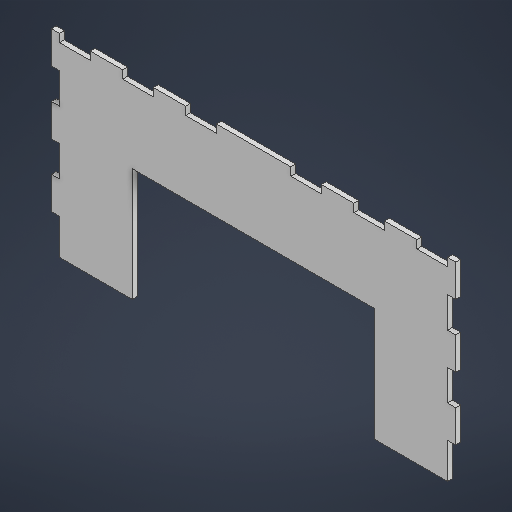
# Autodesk Inventor part: Part1
Saved by Autodesk Inventor 2027.1 (Build 311270010, 270A)
## iProperties
Created: 2026-10-07
Part Number: Part1
Material: Generic
Document SubType Name: Modeling
Designer: daniel
Density: 1 g/cm^3
Appearance: Default
Author: daniel
Autodesk Inventor part; units mm, degrees
ref_plane "YZ Plane" through (0, 0, 0) normal (1, 0, 0) x (0, 1, 0)
ref_plane "XZ Plane" through (0, 0, 0) normal (0, 1, 0) x (-1, 0, 0)
ref_plane "XY Plane" through (0, 0, 0) normal (0, 0, 1) x (1, 0, 0)
sketch "Sketch1" plane through (0, 0, 0) normal (0, 0, 1) x (1, 0, 0)
  line L0 (-39.6936, 53.8926) -> (210.3064, 53.8926)
  line L1 (210.3064, 53.8926) -> (210.3064, -66.1074)
  line L2 (210.3064, -66.1074) -> (-39.6936, -66.1074)
  line L3 (-39.6936, -66.1074) -> (-39.6936, 53.8926)
  line L4 (78.3064, 19.8926) -> (92.3064, 19.8926)
  line L5 (92.3064, 19.8926) -> (92.3064, 14.8926)
  line L6 (92.3064, 14.8926) -> (78.3064, 14.8926)
  line L7 (78.3064, 14.8926) -> (78.3064, 19.8926)
  line L8 (70.3064, 43.8926) -> (75.3064, 43.8926)
  line L9 (75.3064, 43.8926) -> (75.3064, 29.8926)
  line L10 (75.3064, 29.8926) -> (70.3064, 29.8926)
  line L11 (70.3064, 29.8926) -> (70.3064, 43.8926)
  line L12 (95.3064, 43.8926) -> (100.3064, 43.8926)
  line L13 (100.3064, 43.8926) -> (100.3064, 29.8926)
  line L14 (100.3064, 29.8926) -> (95.3064, 29.8926)
  line L15 (95.3064, 29.8926) -> (95.3064, 43.8926)
  line L16 (10.3064, -66.1074) -> (160.3064, -66.1074)
  line L17 (160.3064, -66.1074) -> (160.3064, 3.8926)
  line L18 (160.3064, 3.8926) -> (10.3064, 3.8926)
  line L19 (10.3064, 3.8926) -> (10.3064, -66.1074)
  line L20 (-39.6936, 53.8926) -> (-34.6936, 53.8926)
  line L21 (-34.6936, 53.8926) -> (-34.6936, 33.8926)
  line L22 (-34.6936, 33.8926) -> (-39.6936, 33.8926)
  line L23 (-39.6936, 33.8926) -> (-39.6936, 53.8926)
  line L24 (-39.6936, 33.8926) -> (-34.6936, 33.8926)
  line L25 (-34.6936, 33.8926) -> (-34.6936, 14.8926)
  line L26 (-34.6936, 14.8926) -> (-39.6936, 14.8926)
  line L27 (-39.6936, 14.8926) -> (-39.6936, 33.8926)
  line L28 (-39.6936, 14.8926) -> (-34.6936, 14.8926)
  line L29 (-34.6936, 14.8926) -> (-34.6936, -5.1074)
  line L30 (-34.6936, -5.1074) -> (-39.6936, -5.1074)
  line L31 (-39.6936, -5.1074) -> (-39.6936, 14.8926)
  line L32 (-34.6936, -5.1074) -> (-39.6936, -5.1074)
  line L33 (-39.6936, -5.1074) -> (-39.6936, -24.1074)
  line L34 (-39.6936, -24.1074) -> (-34.6936, -24.1074)
  line L35 (-34.6936, -24.1074) -> (-34.6936, -5.1074)
  line L36 (-39.6936, -24.1074) -> (-34.6936, -24.1074)
  line L37 (-34.6936, -24.1074) -> (-34.6936, -44.1074)
  line L38 (-34.6936, -44.1074) -> (-39.6936, -44.1074)
  line L39 (-39.6936, -44.1074) -> (-39.6936, -24.1074)
  line L40 (-34.6936, -44.1074) -> (-39.6936, -44.1074)
  line L41 (-39.6936, -44.1074) -> (-39.6936, -66.1074)
  line L42 (-39.6936, -66.1074) -> (-34.6936, -66.1074)
  line L43 (-34.6936, -66.1074) -> (-34.6936, -44.1074)
  line L44 (85.3064, 106.0541) -> (85.3064, -171.7507)
  line L45 (210.3064, -66.1074) -> (210.3064, 53.8926)
  line L46 (100.3064, 43.8926) -> (95.3064, 43.8926)
  line L47 (95.3064, 43.8926) -> (95.3064, 29.8926)
  line L48 (95.3064, 29.8926) -> (100.3064, 29.8926)
  line L49 (100.3064, 29.8926) -> (100.3064, 43.8926)
  line L50 (210.3064, 53.8926) -> (205.3064, 53.8926)
  line L51 (205.3064, 53.8926) -> (205.3064, 33.8926)
  line L52 (205.3064, 33.8926) -> (210.3064, 33.8926)
  line L53 (210.3064, 33.8926) -> (210.3064, 53.8926)
  line L54 (210.3064, 33.8926) -> (205.3064, 33.8926)
  line L55 (205.3064, 33.8926) -> (205.3064, 14.8926)
  line L56 (205.3064, 14.8926) -> (210.3064, 14.8926)
  line L57 (210.3064, 14.8926) -> (210.3064, 33.8926)
  line L58 (210.3064, 14.8926) -> (205.3064, 14.8926)
  line L59 (205.3064, 14.8926) -> (205.3064, -5.1074)
  line L60 (205.3064, -5.1074) -> (210.3064, -5.1074)
  line L61 (210.3064, -5.1074) -> (210.3064, 14.8926)
  line L62 (205.3064, -5.1074) -> (210.3064, -5.1074)
  line L63 (210.3064, -5.1074) -> (210.3064, -24.1074)
  line L64 (210.3064, -24.1074) -> (205.3064, -24.1074)
  line L65 (205.3064, -24.1074) -> (205.3064, -5.1074)
  line L66 (210.3064, -24.1074) -> (205.3064, -24.1074)
  line L67 (205.3064, -24.1074) -> (205.3064, -44.1074)
  line L68 (205.3064, -44.1074) -> (210.3064, -44.1074)
  line L69 (210.3064, -44.1074) -> (210.3064, -24.1074)
  line L70 (205.3064, -44.1074) -> (210.3064, -44.1074)
  line L71 (210.3064, -44.1074) -> (210.3064, -66.1074)
  line L72 (210.3064, -66.1074) -> (205.3064, -66.1074)
  line L73 (205.3064, -66.1074) -> (205.3064, -44.1074)
  line L74 (-34.6936, 53.8926) -> (-15.6936, 53.8926)
  line L75 (-15.6936, 53.8926) -> (-15.6936, 48.8926)
  line L76 (-15.6936, 48.8926) -> (-34.6936, 48.8926)
  line L77 (-34.6936, 48.8926) -> (-34.6936, 53.8926)
  line L78 (-15.6936, 48.8926) -> (4.3064, 48.8926)
  line L79 (4.3064, 48.8926) -> (4.3064, 53.8926)
  line L80 (4.3064, 53.8926) -> (-15.6936, 53.8926)
  line L81 (-15.6936, 53.8926) -> (-15.6936, 48.8926)
  line L82 (4.3064, 48.8926) -> (23.3064, 48.8926)
  line L83 (23.3064, 48.8926) -> (23.3064, 53.8926)
  line L84 (23.3064, 53.8926) -> (4.3064, 53.8926)
  line L85 (4.3064, 53.8926) -> (4.3064, 48.8926)
  line L86 (23.3064, 48.8926) -> (43.3064, 48.8926)
  line L87 (43.3064, 48.8926) -> (43.3064, 53.8926)
  line L88 (43.3064, 53.8926) -> (23.3064, 53.8926)
  line L89 (23.3064, 53.8926) -> (23.3064, 48.8926)
  line L90 (43.3064, 48.8926) -> (62.3064, 48.8926)
  line L91 (62.3064, 48.8926) -> (62.3064, 53.8926)
  line L92 (62.3064, 53.8926) -> (43.3064, 53.8926)
  line L93 (43.3064, 53.8926) -> (43.3064, 48.8926)
  line L94 (205.3064, 53.8926) -> (186.3064, 53.8926)
  line L95 (186.3064, 53.8926) -> (186.3064, 48.8926)
  line L96 (186.3064, 48.8926) -> (205.3064, 48.8926)
  line L97 (205.3064, 48.8926) -> (205.3064, 53.8926)
  line L98 (186.3064, 48.8926) -> (166.3064, 48.8926)
  line L99 (166.3064, 48.8926) -> (166.3064, 53.8926)
  line L100 (166.3064, 53.8926) -> (186.3064, 53.8926)
  line L101 (186.3064, 53.8926) -> (186.3064, 48.8926)
  line L102 (166.3064, 48.8926) -> (147.3064, 48.8926)
  line L103 (147.3064, 48.8926) -> (147.3064, 53.8926)
  line L104 (147.3064, 53.8926) -> (166.3064, 53.8926)
  line L105 (166.3064, 53.8926) -> (166.3064, 48.8926)
  line L106 (147.3064, 48.8926) -> (127.3064, 48.8926)
  line L107 (127.3064, 48.8926) -> (127.3064, 53.8926)
  line L108 (127.3064, 53.8926) -> (147.3064, 53.8926)
  line L109 (147.3064, 53.8926) -> (147.3064, 48.8926)
  line L110 (127.3064, 48.8926) -> (108.3064, 48.8926)
  line L111 (108.3064, 48.8926) -> (108.3064, 53.8926)
  line L112 (108.3064, 53.8926) -> (127.3064, 53.8926)
  line L113 (127.3064, 53.8926) -> (127.3064, 48.8926)
  point P0 (0, 0)
  point P1 (92.3064, 17.3926)
  point P2 (75.3064, 36.8926)
  point P3 (95.3064, 36.8926)
  point P4 (97.8064, 43.8926)
  point P5 (72.8064, 43.8926)
  dimension "d0" = 250
  dimension "d1" = 120
  dimension "d2" = 14
  dimension "d3" = 5
  dimension "d4" = 34
  dimension "d5" = 118
  dimension "d6" = 5
  dimension "d7" = 14
  dimension "d8" = 5
  dimension "d9" = 14
  dimension "d10" = 20
  dimension "d11" = 3
  dimension "d12" = 10
  dimension "d13" = 10
  dimension "d14" = 150
  dimension "d15" = 70
  dimension "d16" = 50
  dimension "d17" = 5
  dimension "d18" = 20
  dimension "d19" = 19
  dimension "d20" = 20
  dimension "d21" = 19
  dimension "d22" = 20
  dimension "d25" = 19
  dimension "d26" = 5
  dimension "d27" = 20
  dimension "d28" = 19
  dimension "d29" = 20
  dimension "d30" = 19
  constraints: 228 end point, 32 parallel, 32 symmetric about line, 16 horizontal, 16 perpendicular, 13 point on line, 5 midpoint, 1 vertical
  measures "d0" distance of L1.end L2.end
  measures "d1" distance of L0.end L1.end
  measures "d2" distance of L5.end L6.end
  measures "d3" distance of L4.end L5.end
  measures "d4" distance between parallel lines of L0 L4
  measures "d5" distance from line of L1 point (92.306, 17.393)
  measures "d6" distance of L9.end L10.end
  measures "d7" distance of L8.end L9.end
  measures "d8" distance of L13.end L14.end
  measures "d9" distance of L13.start L13.end
  measures "d10" distance of point (75.306, 36.893) point (95.306, 36.893)
  measures "d11" distance between parallel lines of L7 L9
  measures "d12" distance from line of L0 point (97.806, 43.893)
  measures "d13" distance from line of L0 point (72.806, 43.893)
  measures "d14" distance of L18.end L17.end
  measures "d15" distance of L17.end L16.end
  measures "d16" distance between parallel lines of L1 L17
  measures "d17" distance of L21.end L22.end
  measures "d18" distance of L20.end L21.end
  measures "d19" distance of L24.end L25.end
  measures "d20" distance of L28.end L29.end
  measures "d21" distance of L33.end L32.end
  measures "d22" distance of L36.end L37.end
  measures "d25" distance of L75.end L76.end
  measures "d26" distance of L74.end L75.end
  measures "d27" distance of L80.end L79.end
  measures "d28" distance of L84.end L83.end
  measures "d29" distance of L88.end L87.end
  measures "d30" distance of L92.end L91.end
extrude "Extrusion1" add sketch "Sketch1" along normal blind 3 contours L0 L21 L22 L3 | L0 L79 L78 L75 | L76 L78 L82 L86 L90 L91 L0 L44 L4 L7 L6 L18 L19 L2 L43 L37 L35 L29 L25 L21 | L26 L29 L30 L3 | L0 L87 L86 L83 | L34 L37 L38 L3 | L0 L111 L110 L106 L102 L98 L96 L51 L55 L59 L65 L67 L73 L2 L17 L18 L44 L6 L5 L4 | L44 L6 L7 L4 | L4 L5 L6 L44 | L0 L103 L106 L107 | L0 L95 L98 L99 | L67 L64 L1 L68 | L0 L1 L52 L51 | L59 L56 L1 L60 | L8 L9 L10 L11 | L12 L13 L14 L15
sketch "Sketch2" plane through (0, 0, 0) normal (0, 0, -1) x (-1, 0, 0)
  point P0 (0, 0)
equation "\"d5\" = -0.5 * d2 + 0.5 * d0"
equation "\"d11\" = -0.5 * d2 + 0.5 * d10"
equation "\"d16\" = -0.5 * d14 + 0.5 * d0"
body "Solid1"
